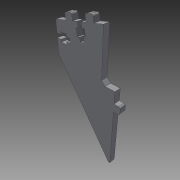
# Autodesk Inventor part: front_panel_brace_middle
Saved by Autodesk Inventor 2014 (Build 180170000, 170)
## iProperties
Created: 2014-03-23
Part Number: front_panel_brace_middle
Material: Plywood, Finish
Document SubType Name: Modeling
Designer: buben
Density: 0.552 g/cm^3
Appearance: Plywood - New
Author: buben
Autodesk Inventor part; units mm, degrees
ref_plane "YZ Plane" through (0, 0, 0) normal (1, 0, 0) x (0, 1, 0)
ref_plane "XZ Plane" through (0, 0, 0) normal (0, 1, 0) x (-1, 0, 0)
ref_plane "XY Plane" through (0, 0, 0) normal (0, 0, 1) x (1, 0, 0)
sketch "Sketch1" plane through (0, 0, 0) normal (0, 1, 0) x (-1, 0, 0)
  line L0 (0, 0) -> (10, 0)
  line L1 (10, 0) -> (66.654, -9.9896)
  line L2 (66.654, -9.9896) -> (66.654, -41.5096)
  line L3 (66.654, -41.5096) -> (2, -133.8451)
  line L4 (2, -133.8451) -> (0, -133.8451)
  line L5 (0, -133.8451) -> (0, 0)
  dimension "d0" = 31.52
  dimension "d1" = 145
  dimension "d2" = 100
  dimension "d3" = 10
  dimension "d4" = 2
  dimension "d5" = 66.654
  constraints: 12 end point, 2 parallel, 1 horizontal, 1 perpendicular
  measures "d0" distance of L1.end L2.end
  measures "d1" angle of L3 L2
  measures "d2" angle of L1 L2
  measures "d3" distance of L0.start L0.end
  measures "d4" distance of L3.end L4.end
  measures "d5" distance between parallel lines of L5 L2
extrude "Extrusion1" add sketch "Sketch1" along normal blind 6.5
sketch "Sketch2" plane through (0, 6.5, 0) normal (0, 1, 0) x (1, 0, 0)
  line L0 (-66.654, 41.5096) -> (-66.654, 9.9896) projected
  line L1 (-66.654, 9.9896) -> (-10, 0) projected
  line L2 (-50.354, 26.3816) -> (-50.354, 21.8816)
  line L3 (-66.654, 21.8816) -> (-66.654, 26.3816)
  line L4 (-61.654, 28.8816) -> (-54.354, 28.8816)
  line L5 (-54.354, 19.3816) -> (-61.654, 19.3816)
  line L6 (-66.654, 26.3816) -> (-61.654, 26.3816)
  line L7 (-54.354, 26.3816) -> (-50.354, 26.3816)
  line L8 (-61.654, 19.3816) -> (-61.654, 21.8816)
  line L9 (-61.654, 26.3816) -> (-61.654, 28.8816)
  line L10 (-50.354, 21.8816) -> (-54.354, 21.8816)
  line L11 (-61.654, 21.8816) -> (-66.654, 21.8816)
  line L12 (-54.354, 28.8816) -> (-54.354, 26.3816)
  line L13 (-54.354, 21.8816) -> (-54.354, 19.3816)
  line L14 (-37.7124, 21.4379) -> (-33.2807, 20.6565)
  line L15 (-36.1112, 4.6041) -> (-40.5428, 5.3855)
  line L16 (-42.1366, 10.7437) -> (-40.869, 17.9328)
  line L17 (-31.5133, 16.2831) -> (-32.7809, 9.094)
  line L18 (-40.5428, 5.3855) -> (-39.6746, 10.3096)
  line L19 (-38.4069, 17.4987) -> (-37.7124, 21.4379)
  line L20 (-32.7809, 9.094) -> (-35.2429, 9.5281)
  line L21 (-39.6746, 10.3096) -> (-42.1366, 10.7437)
  line L22 (-33.2807, 20.6565) -> (-33.9753, 16.7172)
  line L23 (-35.2429, 9.5281) -> (-36.1112, 4.6041)
  line L24 (-40.869, 17.9328) -> (-38.4069, 17.4987)
  line L25 (-33.9753, 16.7172) -> (-31.5133, 16.2831)
  point P0 (-38.327, 4.9948)
  point P1 (-50.354, 24.1316)
  dimension "d8" = 4.5
  dimension "d9" = 5
  dimension "d10" = 4
  dimension "d11" = 7.3
  dimension "d12" = 2.5
  dimension "d13" = 4.5
  dimension "d14" = 5
  dimension "d15" = 4
  dimension "d16" = 7.3
  dimension "d17" = 2.5
  dimension "d35" = 14.142
  constraints: 48 end point, 21 parallel, 12 collinear, 8 perpendicular, 3 horizontal, 3 midpoint
  measures "d8" distance of L2.start L2.end
  measures "d9" distance of L8.end L3.start
  measures "d10" distance of L2.end L10.end
  measures "d11" distance of L5.start L5.end
  measures "d12" distance of L10.end L5.start
  measures "d13" distance of L14.start L14.end
  measures "d14" distance of L20.end L15.start
  measures "d15" distance of L14.end L22.end
  measures "d16" distance of L25.end L17.end
  measures "d17" distance of L22.end L25.end
  measures "d35" vertical distance of L0.end point (-50.354, 24.132)
extrude "Extrusion2" cut sketch "Sketch2" against normal through all
sketch "Sketch3" plane through (0, 6.5, 0) normal (0, 1, 0) x (1, 0, 0)
  line L0 (-66.654, 9.9896) -> (-40.5428, 5.3855) projected
  line L1 (-37.7124, 21.4379) -> (-33.2807, 20.6565) projected
  line L2 (-36.1112, 4.6041) -> (-10, 0) projected
  line L3 (-45.7131, 6.2972) -> (-53.5915, 7.6864)
  line L4 (-53.5915, 7.6864) -> (-54.3729, 3.2547)
  line L5 (-52.7506, 0.9378) -> (-48.8114, 0.2432)
  line L6 (-46.4945, 1.8655) -> (-45.7131, 6.2972)
  line L7 (-30.9409, 3.6925) -> (-23.0625, 2.3033)
  line L8 (-23.0625, 2.3033) -> (-23.8439, -2.1284)
  line L9 (-26.1608, -3.7507) -> (-30.1, -3.0561)
  line L10 (-31.7224, -0.7392) -> (-30.9409, 3.6925)
  arc A0 (-54.3729, 3.2547) -> (-52.7506, 0.9378) centre (-52.4033, 2.9074) ccw
  arc A1 (-48.8114, 0.2432) -> (-46.4945, 1.8655) centre (-48.4641, 2.2128) ccw
  arc A2 (-31.7224, -0.7392) -> (-30.1, -3.0561) centre (-29.7527, -1.0865) ccw
  arc A3 (-26.1608, -3.7507) -> (-23.8439, -2.1284) centre (-25.8135, -1.7811) ccw
  point P0 (-35.4965, 21.0472)
  dimension "d20" = 2
  dimension "d21" = 8
  dimension "d22" = 8
  dimension "d23" = 6.5
  dimension "d24" = 15
  dimension "d25" = 7.5
  constraints: 16 end point, 8 point on circle, 8 tangent, 4 centre point, 4 parallel, 4 point on line, 3 equal radius, 2 perpendicular, 1 collinear, 1 midpoint
  measures "d20" radius of A0
  measures "d21" distance between parallel lines of L6 L4
  measures "d22" distance between parallel lines of L8 L10
  measures "d23" distance between parallel lines of L0 L5
  measures "d24" distance between parallel lines of L10 L6
  measures "d25" distance from line of point (-35.497, 21.047) L6
extrude "Extrusion3" add sketch "Sketch3" against normal blind 6.5
sketch "Sketch4" plane through (0, 6.5, 0) normal (0, 1, 0) x (1, 0, 0)
  line L0 (-23.0625, 2.3033) -> (-10, 0) projected
  line L1 (-10, 0) -> (0, 0) projected
  line L2 (0, 0) -> (0, 133.8451) projected
  line L3 (-61.654, 19.3816) -> (-61.654, 21.8816) projected
  line L4 (0, 50) -> (-10, 50)
  line L5 (-10, 50) -> (-14, 46)
  line L6 (-14, 46) -> (-14, 0.7053)
  dimension "d28" = 45
  dimension "d29" = 10
  dimension "d30" = 50
  dimension "d32" = 4
  constraints: 6 end point, 2 perpendicular, 2 point on line
  measures "d28" angle of L5 L4
  measures "d29" distance of L4.start L4.end
  measures "d30" distance between parallel lines of L1 L4
  measures "d32" horizontal distance of L4.end L5.end
extrude "Extrusion4" cut sketch "Sketch4" against normal through all
sketch "Sketch5" plane through (0, 6.5, 0) normal (0, 1, 0) x (1, 0, 0)
  line L0 (0, 50) -> (0, 133.8451) projected
  line L1 (0, 62.001) -> (4.5, 62.001)
  line L2 (6.5, 64.001) -> (6.5, 68.001)
  line L3 (4.5, 70.001) -> (0, 70.001)
  line L4 (0, 70.001) -> (0, 62.001)
  arc A0 (4.5, 62.001) -> (6.5, 64.001) centre (4.5, 64.001) ccw
  arc A1 (6.5, 68.001) -> (4.5, 70.001) centre (4.5, 68.001) ccw
  point P0 (0, 0)
  dimension "d36" = 2
  dimension "d37" = 8
  dimension "d38" = 6.5
  dimension "d39" = 12.001
  constraints: 8 end point, 4 point on circle, 4 tangent, 2 centre point, 2 parallel, 1 equal radius, 1 horizontal, 1 perpendicular, 1 point on line
  measures "d36" radius of A0
  measures "d37" distance between parallel lines of L1 L3
  measures "d38" distance between parallel lines of L2 L0
  measures "d39" distance from line of L0.start L1
extrude "Extrusion5" add sketch "Sketch5" against normal blind 6.5
equation "\"d25\" = 0.5 * d24"
body "Solid1"
